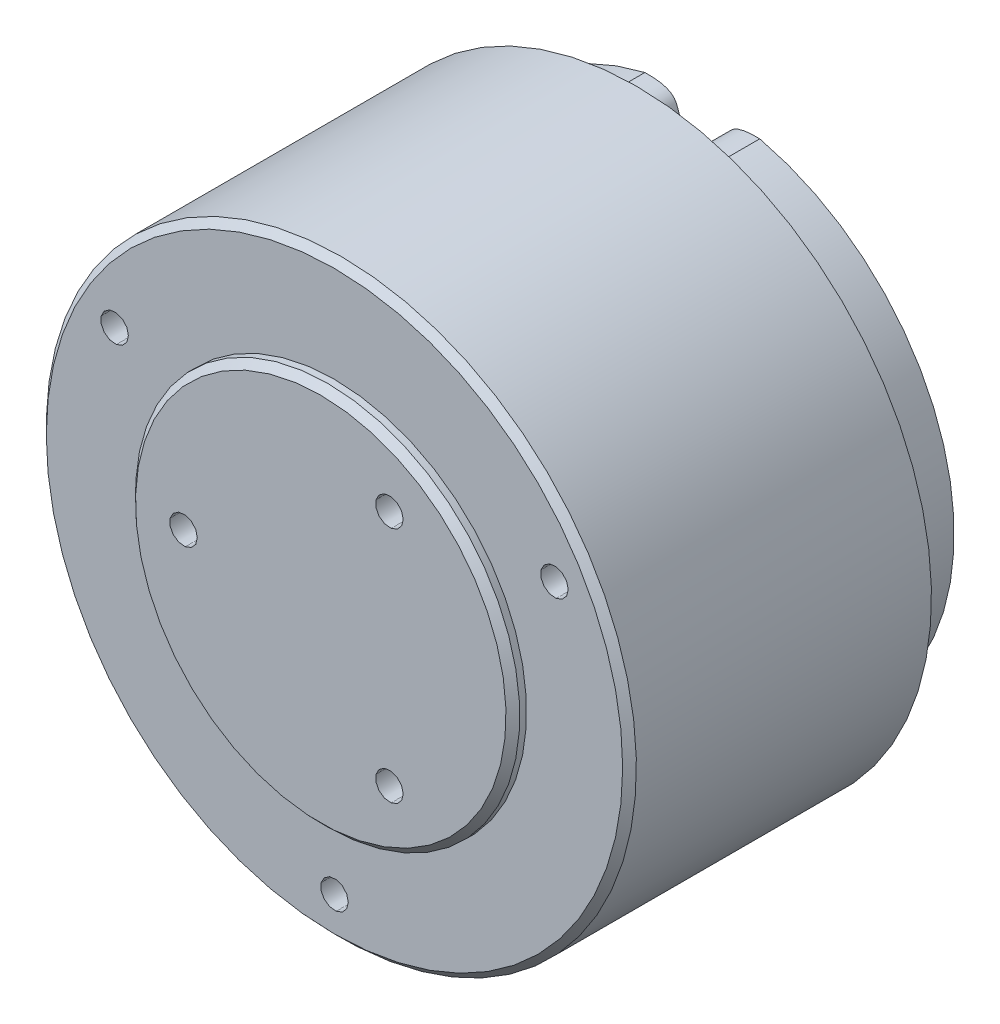
# Autodesk Inventor part: GIM3505-8_with-driver
Saved by Autodesk Inventor 2024 (Build 280153000, 153)
## iProperties
Created: 2024-11-12
Part Number: GIM3505-8_with-driver
Material: Generic
Document SubType Name: Modeling
Designer: kiyo
Density: 2.67168 g/cm^3
Appearance: 滑らか - 黒
Mass: 97 g
Surface Area: 87.4179 cm^2
Volume: 36.3067 cm^3
Author: kiyo
Autodesk Inventor part; units mm, degrees
ref_plane "YZ Plane" through (0, 0, 0) normal (1, 0, 0) x (0, 1, 0)
ref_plane "XZ Plane" through (0, 0, 0) normal (0, 1, 0) x (-1, 0, 0)
ref_plane "XY Plane" through (0, 0, 0) normal (0, 0, 1) x (1, 0, 0)
sketch "スケッチ1" plane through (0, 0, 0) normal (1, 0, 0) x (0, 1, 0)
  line L0 (0, 11.5) -> (0, -11.5)
  line L1 (0, -11.5) -> (21.5, -11.5)
  line L2 (21.5, -11.5) -> (21.5, 10)
  line L3 (21.5, 10) -> (21, 10.5)
  line L4 (21, 10.5) -> (14, 10.5)
  line L5 (14, 10.5) -> (14, 11)
  line L6 (14, 11) -> (13.5, 11.5)
  line L7 (13.5, 11.5) -> (0, 11.5)
  line L8 (0, 11.5) -> (0, -28.8949)
  line L9 (18.35, -12.5) -> (0, -12.5)
  line L10 (0, -12.5) -> (0, -16.3)
  line L11 (0, -16.3) -> (18.35, -16.3)
  line L12 (18.35, -16.3) -> (18.35, -12.5)
  point P0 (0, 0)
  point P1 (0, -12.5)
  dimension "d0" = 23
  dimension "d1" = 21.5
  dimension "d5" = 0.5
  dimension "d6" = 21
  dimension "d7" = 0.5
  dimension "d8" = 1
  dimension "d36" = 1
  dimension "d37" = 3.8
  dimension "d38" = 18.35
  dimension "d40" = 14
  constraints: 26 end point, 5 parallel, 3 perpendicular, 2 midpoint, 2 vertical, 1 collinear, 1 horizontal
  measures "d0" distance of L0.start L0.end
  measures "d1" distance between parallel lines of L0 L2
  measures "d5" distance from line of L2.end L4
  measures "d6" horizontal distance of L0.start L3.end
  measures "d7" distance of L4.end L5.end
  measures "d8" distance between parallel lines of L7 L4
  measures "d36" distance between parallel lines of L1 L9
  measures "d37" distance of L11.end L9.start
  measures "d38" distance of L10.end L11.end
  measures "d40" distance between parallel lines of L8 L5
revolve "回転1" add sketch "スケッチ1" angle 360 about axis through (0, 0, 11.5) along (0, 0, -1)
sketch "スケッチ2" plane through (0, 0, 11.5) normal (0, 0, 1) x (1, 0, 0)
  circle A0 centre (0, 0) radius 13.5 projected
  point P0 (0, 0)
  point P1 (-10, 0)
  point P2 (5, -8.6603)
  point P3 (5, 8.6603)
  dimension "d10" = 10
  dimension "d11" = 0
  dimension "d14" = 360
  constraints: 4 other
  measures "d10" distance of point (0, 0) point (-10, 0)
  measures "d11" vertical distance of point (0, 0) point (-10, 0)
hole "穴1" at (-10, 0, 11.5) at (5, -8.6603, 11.5) at (5, 8.6603, 11.5) direction (0, 0, -1) diameter 2.013 depth 4 tip angle 118 thread size "M2.5x0.45" designation "M2.5" class "6H" standard "GB Metric profile"
sketch "スケッチ3" plane through (0, 0, 10.5) normal (0, 0, 1) x (1, 0, 0)
  circle A0 centre (0, 0) radius 21 projected
  circle A1 centre (0, 0) radius 18.5
  point P0 (0, 0)
  point P1 (0, -18.5)
  point P2 (16.0215, 9.25)
  point P3 (-16.0215, 9.25)
  dimension "d23" = 37
  dimension "d24" = 0
  dimension "d27" = 360
  constraints: 1 coincident, 1 vertical alignment, 6 other
  measures "d24" horizontal distance of point (0, 0) point (0, -18.5)
hole "穴2" at (0, -18.5, 10.5) at (16.0215, 9.25, 10.5) at (-16.0215, 9.25, 10.5) direction (0, 0, -1) diameter 2.013 depth 5 tip angle 118 thread size "M2.5x0.45" designation "M2.5" class "6H" standard "GB Metric profile"
sketch "スケッチ4" plane through (0, 0, -11.5) normal (0, 0, -1) x (-1, 0, 0)
  circle A0 centre (0, 0) radius 19.6
  line L0 (0, 0) -> (0, -21.5)
  circle A1 centre (0, 0) radius 21.5 projected
  line L1 (0, 0) -> (-13.8593, -13.8593)
  point P0 (0, -17.5)
  point P1 (0, 17.5)
  point P2 (13.8593, -13.8593)
  point P3 (13.8593, 13.8593)
  point P4 (-13.8593, 13.8593)
  dimension "d45" = 39.2
  dimension "d41" = 35
  dimension "d42" = 0
  dimension "d43" = 0
  dimension "d44" = 17.5
  dimension "d46" = 45
  dimension "d49" = 360
  constraints: 4 end point, 2 coincident, 1 vertical, 1 vertical alignment, 9 other
  measures "d41" distance of point (0, -17.5) point (0, 17.5)
  measures "d42" horizontal distance of point (0, 0) point (0, -17.5)
  measures "d43" horizontal distance of point (0, 0) point (0, 17.5)
  measures "d44" distance of point (0, 0) point (0, 17.5)
  measures "d46" angle of L0 L1
hole "穴3" at (13.8593, -13.8593, -11.5) at (-13.8593, -13.8593, -11.5) at (-13.8593, 13.8593, -11.5) at (13.8593, 13.8593, -11.5) direction (0, 0, 1) diameter 2.013 depth 4 tip angle 118 thread size "M2.5x0.45" designation "M2.5" class "6H" standard "GB Metric profile"
hole "穴4" at (0, -17.5, -11.5) at (0, 17.5, -11.5) direction (0, 0, 1) diameter 1.567 depth 4 tip angle 118 thread size "M2x0.4" designation "M2" class "6H" standard "GB Metric profile"
sketch "スケッチ5" plane through (0, 0, -16.3) normal (0, 0, -1) x (-1, 0, 0)
  circle A0 centre (0, 0) radius 18.35 projected
  spline S0 degree 3 poles (4.1841, -17.8666) (0.2456, -17.9761) (2.9714, -15.4318) (0, -15.1735) knots 0 0 0 0 1 1 1 1
  line L0 (0, -15.1735) -> (0, -18.35)
  spline S1 degree 3 poles (-4.1841, -17.8666) (-0.2456, -17.9761) (-2.9714, -15.4318) (0, -15.1735) knots 0 0 0 0 1 1 1 1
  line L1 (0, 0) -> (-18.35, 0)
  spline S2 degree 3 poles (4.1841, 17.8666) (0.2456, 17.9761) (2.9714, 15.4318) (0, 15.1735) knots 0 0 0 0 1 1 1 1
  spline S3 degree 3 poles (-4.1841, 17.8666) (-0.2456, 17.9761) (-2.9714, 15.4318) (0, 15.1735) knots 0 0 0 0 1 1 1 1
  point P0 (0, 0)
  point P1 (1.867, -17.0431)
  point P2 (1.537, -16.0265)
  point P3 (-1.867, -17.0431)
  point P4 (-1.537, -16.0265)
  point P5 (1.867, 17.0431)
  point P6 (1.537, 16.0265)
  point P7 (-1.867, 17.0431)
  point P8 (-1.537, 16.0265)
  point P9 (-4.1841, 17.8666)
  point P10 (4.1841, 17.8666)
  point P11 (-4.1841, -17.8666)
  constraints: 10 symmetric about line, 4 end point, 3 point on circle, 1 horizontal, 1 vertical, 16 other
extrude "押し出し1" cut sketch "スケッチ5" against normal blind 3.8 contours S2 S3 A0 | A0 L0 S0 | A0 S1 L0
